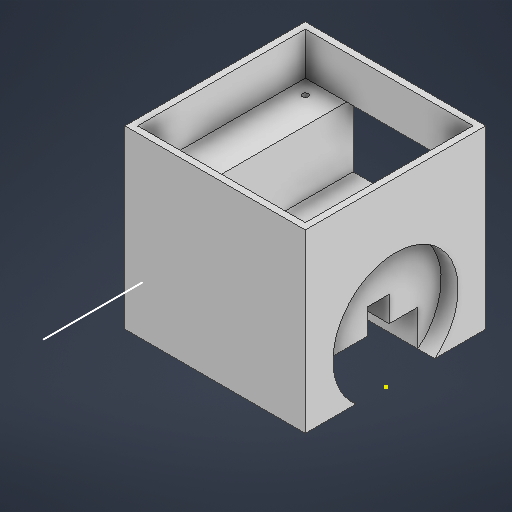
# Autodesk Inventor part: RobotBase
Saved by Autodesk Inventor 2026.2 (Build 302298000, 298)
## iProperties
Created: 2026-09-23
Part Number: RobotBase
Material: Generic
Document SubType Name: Modeling
Designer: Brian Wang
Density: 1 g/cm^3
Appearance: Default
Author: Brian Wang
Autodesk Inventor part; units mm, degrees
ref_plane "YZ Plane" through (0, 0, 0) normal (1, 0, 0) x (0, 1, 0)
ref_plane "XZ Plane" through (0, 0, 0) normal (0, 1, 0) x (-1, 0, 0)
ref_plane "XY Plane" through (0, 0, 0) normal (0, 0, 1) x (1, 0, 0)
sketch "Sketch1" plane through (0, 0, 0) normal (0, 1, 0) x (-1, 0, 0)
  line L0 (32.6686, 38.0315) -> (-52.3314, 38.0315)
  line L1 (-52.3314, 38.0315) -> (-52.3314, -46.9685)
  line L2 (-52.3314, -46.9685) -> (32.6686, -46.9685)
  line L3 (32.6686, -46.9685) -> (32.6686, 38.0315)
  point P0 (0, 0)
  dimension "d0" = 85
  dimension "d1" = 85
  constraints: 8 end point, 2 parallel, 1 horizontal, 1 perpendicular
  measures "d0" distance of L2.end L1.end
  measures "d1" distance of L1.end L0.end
extrude "Extrusion1" add sketch "Sketch1" along normal blind 73
sketch "Sketch2" plane through (52.3314, 0, 38.0315) normal (1, 0, 0) x (0, 0, -1)
  point P0 (38.0315, 0)
sketch "Sketch3" plane through (52.3314, 0, 38.0315) normal (1, 0, 0) x (0, 0, -1)
  circle A0 centre (42.5, 23) radius 29.5
  line L0 (0, 73) -> (85, 73) projected
  line L1 (85, 0) -> (85, 73) projected
  point P0 (38.0315, 0)
  dimension "d4" = 59
  dimension "d5" = 50
  dimension "d6" = 42.5
  constraints: 1 centre point
  measures "d4" diameter of A0
  measures "d5" distance from line of L0 A0.centre
  measures "d6" distance from line of L1 A0.centre
extrude "Extrusion2" cut sketch "Sketch3" against normal blind 8
sketch "Sketch4" plane through (-32.6686, 0, -46.9685) normal (-1, 0, 0) x (0, 0, 1)
  arc A0 (60.973, 0) -> (24.027, 0) centre (42.5, 23) ccw projected
  circle A1 centre (42.5, 23) radius 29.5
  point P0 (46.9685, 0)
  point P1 (24.027, 0)
  constraints: 1 centre point, 1 coincident
extrude "Extrusion3" cut sketch "Sketch4" against normal blind 8
sketch "Sketch5" plane through (0, 0, 0) normal (0, -1, 0) x (1, 0, 0)
  line L0 (-24.6686, 14.0044) -> (-24.6686, -22.9415) projected
  line L1 (-24.6686, -9.4685) -> (5.3314, -9.4685)
  line L2 (5.3314, -9.4685) -> (5.3314, 0.5315)
  line L3 (-4.6686, 0.5315) -> (-24.6686, 0.5315)
  line L4 (-24.6686, 0.5315) -> (-24.6686, -9.4685)
  line L5 (-4.6686, 0.5315) -> (-4.6686, 25.5315)
  line L6 (-4.6686, 25.5315) -> (5.3314, 25.5315)
  line L7 (5.3314, 25.5315) -> (5.3314, 0.5315)
  line L8 (-24.6686, -9.4685) -> (-24.6686, 0.5315)
  line L9 (44.3314, -9.4685) -> (14.3314, -9.4685)
  line L10 (14.3314, -9.4685) -> (14.3314, 0.5315)
  line L11 (24.1898, 0.5315) -> (44.3314, 0.5315)
  line L12 (24.1898, 0.5315) -> (24.3314, 25.5315)
  line L13 (24.3314, 25.5315) -> (14.3314, 25.5315)
  line L14 (14.3314, 25.5315) -> (14.3314, 0.5315)
  line L15 (44.3314, -9.4685) -> (44.3314, 0.5315)
  line L16 (44.3314, -22.9415) -> (44.3314, 14.0044) projected
  point P0 (0, 0)
  dimension "d13" = 13.473
  dimension "d35" = 10
  dimension "d36" = 9
  dimension "d37" = 10
  constraints: 30 end point, 3 parallel, 2 collinear, 1 horizontal, 1 perpendicular, 1 point on line, 1 vertical
  measures "d13" distance from line of L0.end L1
  measures "d35" distance of L12.end L13.end
  measures "d36" distance between parallel lines of L14 L7
  measures "d37" distance of L5.end L6.end
sketch "Sketch6" plane through (-24.6686, 0, -46.9685) normal (-1, 0, 0) x (0, 0, 1)
  arc A0 (60.973, 0) -> (24.027, 0) centre (42.5, 23) ccw projected
  line L0 (42.5, 23) -> (131.4973, 23)
  point P0 (46.9685, 0)
  constraints: 2 end point, 1 horizontal
extrude "Extrusion4" cut sketch "Sketch5" against normal blind 29
sketch "Sketch7" plane through (0, 0, 0) normal (0, -1, 0) x (1, 0, 0)
  line L0 (-24.6686, -22.9415) -> (44.3314, -22.9415)
  line L1 (44.3314, -22.9415) -> (44.3314, 31.0585)
  line L2 (44.3314, 31.0585) -> (-24.6686, 31.0585)
  line L3 (-24.6686, 31.0585) -> (-24.6686, -22.9415)
  point P0 (0, 0)
  dimension "d19" = 69
  dimension "d20" = 54
  constraints: 8 end point, 2 parallel, 1 horizontal, 1 perpendicular
  measures "d19" distance of L2.end L1.end
  measures "d20" distance of L1.end L0.end
extrude "Extrusion5" cut sketch "Sketch7" against normal blind 17
sketch "Sketch8" plane through (0, 17, 0) normal (0, -1, 0) x (1, 0, 0)
  circle A0 centre (-15.6686, -13.9415) radius 2
  circle A1 centre (-15.6686, 11.0585) radius 2
  circle A2 centre (34.3314, 11.0585) radius 2
  circle A3 centre (34.3314, -13.9415) radius 2
  line L0 (-26.1879, -23.917) -> (41.8121, -23.917)
  line L1 (-24.6686, 31.0585) -> (44.3314, 31.0585) projected
  line L2 (-24.6686, 31.0585) -> (44.3314, 31.0585)
  line L3 (44.3314, 31.0585) -> (44.3314, -22.9415)
  line L4 (44.3314, -22.9415) -> (-24.6686, -22.9415)
  line L5 (-24.6686, -22.9415) -> (-24.6686, 31.0585)
  point P0 (0, 0)
  point P1 (-18.7833, -12.5016)
  dimension "d23" = 4
  dimension "d24" = 4
  dimension "d25" = 4
  dimension "d26" = 4
  dimension "d27" = 50
  dimension "d28" = 25
  dimension "d31" = 9
  dimension "d32" = 9
  constraints: 10 end point, 4 centre point, 2 horizontal alignment, 2 parallel, 2 vertical alignment, 1 horizontal, 1 perpendicular
  measures "d23" diameter of A0
  measures "d24" diameter of A1
  measures "d25" diameter of A2
  measures "d26" diameter of A3
  measures "d27" distance of A3.centre A0.centre
  measures "d28" distance of A1.centre A0.centre
  measures "d31" distance from line of L5 A0.centre
  measures "d32" distance from line of L4 A0.centre
extrude "Extrusion6" cut sketch "Sketch8" against normal blind 10 contours A0 | A1 | A2 | A3
sketch "Sketch9" plane through (0, 29, 0) normal (0, -1, 0) x (1, 0, 0)
  line L0 (24.1898, 0.5315) -> (24.3314, 25.5315) projected
  line L1 (14.3314, 25.5315) -> (14.3314, -9.4685) projected
  line L2 (24.3314, 25.5315) -> (14.3314, 25.5315)
  line L3 (14.3314, 25.5315) -> (14.3314, 19.5315)
  line L4 (14.3314, 19.5315) -> (24.3314, 19.5315)
  line L5 (24.3314, 19.5315) -> (24.3314, 25.5315)
  line L6 (5.3314, -9.4685) -> (5.3314, 25.5315) projected
  line L7 (5.3314, 25.5315) -> (-14.6686, 25.5315)
  line L8 (-14.6686, 25.5315) -> (-14.6686, 19.5315)
  line L9 (-14.6686, 19.5315) -> (5.3314, 19.5315)
  line L10 (5.3314, 19.5315) -> (5.3314, 25.5315)
  point P0 (0, 0)
  point P1 (24.2974, 19.5315)
  dimension "d39" = 20
  dimension "d40" = 6
  dimension "d47" = 10
  constraints: 16 end point, 2 horizontal, 2 parallel, 2 perpendicular, 1 point on line
  measures "d39" distance of L9.end L8.end
  measures "d40" distance of L8.end L7.end
  measures "d47" distance of L3.end L4.end
extrude "Extrusion7" cut sketch "Sketch9" against normal blind 61.25 contours L4 L1 L2 L0 | L9 L8 L7 L6
sketch "Sketch10" plane through (0, 73, 0) normal (0, 1, 0) x (1, 0, 0)
  line L0 (52.3314, 46.9685) -> (-32.6686, 46.9685) projected
  line L1 (-10.1686, 46.9685) -> (29.8314, 46.9685)
  line L2 (29.8314, 46.9685) -> (29.8314, -35.0315)
  line L3 (29.8314, -35.0315) -> (-10.1686, -35.0315)
  line L4 (-10.1686, -35.0315) -> (-10.1686, 46.9685)
  line L5 (-32.6686, 46.9685) -> (-32.6686, -38.0315) projected
  point P0 (0, 0)
  dimension "d43" = 40
  dimension "d44" = 82
  dimension "d51" = 22.5
  constraints: 8 end point, 2 parallel, 1 horizontal, 1 perpendicular, 1 point on line
  measures "d43" distance of L2.end L3.end
  measures "d44" distance of L1.end L2.end
  measures "d51" distance between parallel lines of L5 L4
sketch "Sketch11" plane through (0, 29, 0) normal (0, -1, 0) x (1, 0, 0)
  line L0 (24.2974, 19.5315) -> (14.3314, 19.5315) projected
  line L1 (14.3314, 19.5315) -> (34.3314, 19.5315)
  line L2 (34.3314, 19.5315) -> (34.3314, 25.5315)
  line L3 (34.3314, 25.5315) -> (14.3314, 25.5315)
  line L4 (14.3314, 25.5315) -> (14.3314, 19.5315)
  point P0 (0, 0)
  dimension "d48" = 20
  constraints: 8 end point, 2 parallel, 1 horizontal, 1 perpendicular
  measures "d48" distance of L3.end L2.end
extrude "Extrusion8" cut sketch "Sketch11" against normal blind 61.25
extrude "Extrusion9" cut sketch "Sketch10" against normal blind 40
sketch "Sketch12" plane through (0, 73, 0) normal (0, 1, 0) x (1, 0, 0)
  line L0 (-56.5689, -78.065) -> (64.3856, -78.065)
  line L1 (64.3856, -78.065) -> (64.3856, 116.3261)
  line L2 (64.3856, 116.3261) -> (-56.5689, 116.3261)
  line L3 (-56.5689, 116.3261) -> (-56.5689, -78.065)
  point P0 (0, 0)
  constraints: 8 end point, 2 parallel, 1 horizontal, 1 perpendicular
extrude "Extrusion10" cut sketch "Sketch12" against normal blind 10
sketch "Sketch14" plane through (0, 63, 0) normal (0, 1, 0) x (1, 0, 0)
  circle A0 centre (42.3314, -28.0315) radius 1.385
  circle A1 centre (-22.6686, -28.0315) radius 1.385
  circle A2 centre (-22.6686, 36.9685) radius 1.385
  circle A3 centre (42.3314, 36.9685) radius 1.385
  line L0 (52.3314, 46.9685) -> (52.3314, -38.0315) projected
  line L1 (52.3314, -38.0315) -> (-32.6686, -38.0315) projected
  line L2 (-32.6686, -38.0315) -> (-32.6686, 46.9685) projected
  point P0 (0, 0)
  dimension "d56" = 2.77
  dimension "d57" = 2.77
  dimension "d58" = 2.77
  dimension "d59" = 2.77
  dimension "d60" = 65
  dimension "d61" = 65
  dimension "d62" = 10
  dimension "d63" = 10
  dimension "d64" = 10
  constraints: 4 centre point, 2 horizontal alignment, 1 vertical alignment
  measures "d56" diameter of A0
  measures "d57" diameter of A1
  measures "d58" diameter of A2
  measures "d59" diameter of A3
  measures "d60" distance of A3.centre A0.centre
  measures "d61" distance of A1.centre A0.centre
  measures "d62" distance from line of L0 A0.centre
  measures "d63" distance from line of L1 A0.centre
  measures "d64" distance from line of L2 A2.centre
extrude "Extrusion11" cut sketch "Sketch14" against normal blind 10
sketch "Sketch15" plane through (0, 63, 0) normal (0, 1, 0) x (1, 0, 0)
  line L0 (-32.6686, 46.9685) -> (-32.6686, 22.9415) projected
  line L1 (-32.6686, 46.9685) -> (-29.6686, 46.9685)
  line L2 (52.3314, 46.9685) -> (-32.6686, 46.9685) projected
  line L3 (-29.6686, 43.9685) -> (-29.6686, -35.0315)
  line L4 (-32.6686, -38.0315) -> (-32.6686, 46.9685) projected
  line L5 (-32.6686, -38.0315) -> (-29.6686, -38.0315)
  line L6 (-29.6686, 46.9685) -> (-32.6686, 46.9685)
  line L7 (-32.6686, 46.9685) -> (-32.6686, -38.0315)
  line L8 (52.3314, 46.9685) -> (52.3314, -38.0315) projected
  line L9 (52.3314, -38.0315) -> (-29.6686, -38.0315)
  line L10 (-29.6686, -35.0315) -> (49.3314, -35.0315)
  line L11 (52.3314, -35.0315) -> (52.3314, -38.0315)
  line L12 (52.3314, 46.9685) -> (49.3314, 46.9685)
  line L13 (49.3314, 43.9685) -> (49.3314, -35.0315)
  line L14 (49.3314, -38.0315) -> (52.3314, -38.0315)
  line L15 (52.3314, -38.0315) -> (52.3314, 46.9685)
  line L16 (49.3314, 46.9685) -> (-29.6686, 46.9685)
  line L17 (-29.6686, 43.9685) -> (49.3314, 43.9685)
  point P0 (0, 0)
  dimension "d67" = 3
  dimension "d69" = 3
  dimension "d70" = 3
  constraints: 28 end point, 5 parallel, 4 horizontal, 2 perpendicular, 2 point on line
  measures "d67" distance of L0.start L1.end
  measures "d69" distance of L14.end L14.start
  measures "d70" distance of L3.start L16.end
extrude "Extrusion12" add sketch "Sketch15" along normal blind 20
sketch "Sketch16" plane through (0, 29, 0) normal (0, 1, 0) x (1, 0, 0)
  line L0 (-14.6686, -25.5315) -> (-14.6686, -19.5315) projected
  line L1 (5.3314, 9.4685) -> (5.3314, -25.5315) projected
  line L2 (-14.6686, -19.5315) -> (5.3314, -19.5315)
  line L3 (5.3314, -19.5315) -> (5.3314, -25.5315)
  line L4 (5.3314, -25.5315) -> (-14.6686, -25.5315)
  line L5 (-14.6686, -25.5315) -> (-14.6686, -19.5315)
  line L6 (24.2974, -19.5315) -> (14.3314, -19.5315) projected
  line L7 (34.3314, -25.5315) -> (24.3314, -25.5315) projected
  line L8 (14.3314, -19.5315) -> (34.3314, -19.5315)
  line L9 (34.3314, -19.5315) -> (34.3314, -25.5315)
  line L10 (34.3314, -25.5315) -> (14.3314, -25.5315)
  line L11 (14.3314, -25.5315) -> (14.3314, -19.5315)
  point P0 (0, 0)
  point P1 (5.3314, -19.5315)
  constraints: 16 end point, 4 parallel, 2 horizontal, 2 perpendicular
extrude "Extrusion13" cut sketch "Sketch16" against normal through all
sketch "Sketch17" plane through (0, 0, 0) normal (0, -1, 0) x (1, 0, 0)
  point P0 (0, 0)
sketch "Sketch18" plane through (0, 17, 0) normal (0, -1, 0) x (1, 0, 0)
  line L0 (5.3314, 19.5315) -> (5.3314, -9.4685) projected
  line L1 (5.3314, -9.4685) -> (16.5671, -9.4685)
  line L2 (16.5671, -9.4685) -> (16.5671, 0.5747)
  line L3 (16.5671, 0.5747) -> (5.3314, 0.5747)
  line L4 (5.3314, 0.5747) -> (5.3314, -9.4685)
  point P0 (0, 0)
  constraints: 8 end point, 2 parallel, 1 horizontal, 1 perpendicular
body "Solid1"
